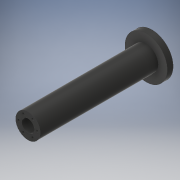
# Autodesk Inventor part: TA03
Saved by Autodesk Inventor 2017 (Build 210142000, 142)
## iProperties
Created: 2018-10-09
Part Number: TA03
Material: ABS Plastic
Document SubType Name: Modeling
Designer: Zach
Density: 1.06 g/cm^3
Appearance: Smooth - Black
Author: Zach
Autodesk Inventor part; units mm, degrees
ref_plane "YZ Plane" through (0, 0, 0) normal (1, 0, 0) x (0, 1, 0)
ref_plane "XZ Plane" through (0, 0, 0) normal (0, 1, 0) x (-1, 0, 0)
ref_plane "XY Plane" through (0, 0, 0) normal (0, 0, 1) x (1, 0, 0)
sketch "Sketch1" plane through (0, 0, 0) normal (0, 0, 1) x (1, 0, 0)
  circle A0 centre (0, 0) radius 7.5
  circle A1 centre (0, 0) radius 14.5
  dimension "d0" = 15
  dimension "d1" = 29
  constraints: 2 centre point, 2 coincident
  measures "d0" diameter of A0
  measures "d1" diameter of A1
extrude "Extrusion1" add sketch "Sketch1" along normal blind 140
sketch "Sketch2" plane through (0, 0, 0) normal (0, 0, -1) x (-1, 0, 0)
  circle A0 centre (0, 0) radius 25
  circle A1 centre (0, 0) radius 7.5 projected
  dimension "d4" = 50
  constraints: 1 centre point, 1 coincident
  measures "d4" diameter of A0
extrude "Extrusion2" add sketch "Sketch2" along normal blind 7
sketch "Sketch3" plane through (0, 0, 140) normal (0, 0, 1) x (1, 0, 0)
  circle A0 centre (11, 0) radius 1.5
  circle A1 centre (0, 0) radius 7.5 projected
  line L0 (7.5, 0) -> (14.5, 0) construction
  circle A2 centre (0, 0) radius 14.5 projected
  line L1 (3.75, 6.4952) -> (7.25, 12.5574) construction
  circle A3 centre (5.5, 9.5263) radius 1.5
  line L2 (-3.75, 6.4952) -> (-7.25, 12.5574) construction
  circle A4 centre (-5.5, 9.5263) radius 1.5
  line L3 (-7.5, 0) -> (-14.5, 0) construction
  circle A5 centre (-11, 0) radius 1.5
  line L4 (-3.75, -6.4952) -> (-7.25, -12.5574) construction
  circle A6 centre (-5.5, -9.5263) radius 1.5
  line L5 (3.75, -6.4952) -> (7.25, -12.5574) construction
  circle A7 centre (5.5, -9.5263) radius 1.5
  dimension "d7" = 3
  dimension "d10" = 360
  constraints: 12 end point, 6 centre point, 6 coincident, 3 horizontal alignment, 1 horizontal, 1 midpoint, 39 other
  measures "d7" diameter of A0
extrude "Extrusion3" cut sketch "Sketch3" against normal blind 25 contours A0 | A3 | A4 | A5 | A6 | A7
body "Solid1"
